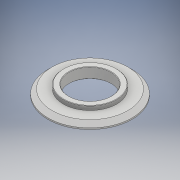
# Autodesk Inventor part: KMB601機械油封墊片(T=7.5-外徑60)
Saved by Autodesk Inventor 2018 (Build 220112000, 112)
## iProperties
Created: 2025-03-12
Part Number: KMB601機械油封墊片(T=7.5-外徑60)
Material: 一般
Document SubType Name: Modeling
Designer: User
Density: 1 g/cm^3
Appearance: 預設
Author: User
Autodesk Inventor part; units mm, degrees
ref_plane "YZ Plane" through (0, 0, 0) normal (1, 0, 0) x (0, 1, 0)
ref_plane "XZ Plane" through (0, 0, 0) normal (0, 1, 0) x (-1, 0, 0)
ref_plane "XY Plane" through (0, 0, 0) normal (0, 0, 1) x (1, 0, 0)
sketch "草圖1" plane through (0, 0, 0) normal (0, 0, 1) x (1, 0, 0)
  circle A0 centre (0, 0) radius 30
  circle A1 centre (0, 0) radius 15
  dimension "d0" = 60
  dimension "d1" = 30
  constraints: 2 centre point, 2 coincident
  measures "d0" diameter of A0
  measures "d1" diameter of A1
extrude "擠出1" add sketch "草圖1" along normal blind 7.5
sketch "草圖2" plane through (0, 0, 0) normal (0, 0, -1) x (-1, 0, 0)
  circle A0 centre (0, 0) radius 20
  circle A1 centre (0, 0) radius 34.9484
  dimension "d4" = 40
  constraints: 2 centre point, 2 coincident
  measures "d4" diameter of A0
extrude "擠出2" cut sketch "草圖2" against normal blind 0.5
sketch "草圖3" plane through (0, 0, 7.5) normal (0, 0, 1) x (1, 0, 0)
  circle A0 centre (0, 0) radius 19
  circle A1 centre (0, 0) radius 30.8877
  dimension "d7" = 38
  constraints: 2 centre point, 2 coincident
  measures "d7" diameter of A0
extrude "擠出3" cut sketch "草圖3" against normal blind 3
chamfer "倒角1" distance 3 angle 45 1 edges at (-30, 0, 4.5)
chamfer "倒角2" distance 0.3 angle 45 2 edges at (-15, 0, 7.5) (-19, 0, 7.5)
chamfer "倒角3" distance 0.3 angle 45 1 edges at (-15, 0, 0)
